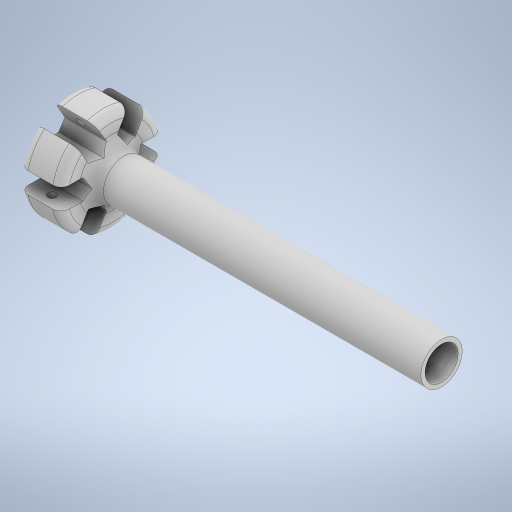
# Autodesk Inventor part: tija_suport
Saved by Autodesk Inventor 2024.2 (Build 282272000, 272)
## iProperties
Created: 2024-03-13
Part Number: tija_suport
Material: Genérico
Document SubType Name: Modeling
Designer: riera
Density: 1 g/cm^3
Appearance: Valor por defecto
Author: riera
Autodesk Inventor part; units mm, degrees
ref_plane "YZ Plane" through (0, 0, 0) normal (1, 0, 0) x (0, 1, 0)
ref_plane "XY Plane" through (0, 0, 0) normal (0, 0, 1) x (1, 0, 0)
sketch "Boceto1" plane through (0, 0, 0) normal (1, 0, 0) x (0, 1, 0)
  circle A0 centre (0, 0) radius 12.5
  dimension "d0" = 25
  constraints: 1 centre point, 1 coincident
  measures "d0" diameter of A0
extrude "Extrusión1" add sketch "Boceto1" along normal blind 10
sketch "Boceto2" plane through (10, 0, 0) normal (1, 0, 0) x (0, 0, -1)
  circle A0 centre (0, 0) radius 5
  circle A1 centre (0, 0) radius 4
  dimension "d3" = 10
  dimension "d35" = 8
  constraints: 2 centre point, 2 coincident
  measures "d3" diameter of A0
  measures "d35" diameter of A1
extrude "Extrusión2" add sketch "Boceto2" along normal blind 80
sketch "Boceto3" plane through (0, 0, 0) normal (-1, 0, 0) x (0, 0, 1)
  circle A0 centre (0, 0) radius 12.5 projected
  line L0 (6.9974, 2.5) -> (5.7474, 0)
  line L1 (5.7474, 0) -> (6.9974, -2.5)
  line L2 (0, 0) -> (0, 7.6455)
  line L3 (6.9974, 2.5) -> (12.5, 2.5)
  line L4 (6.9974, -2.5) -> (12.5, -2.5)
  line L5 (12.5, -2.5) -> (12.5, 2.5)
  dimension "d9" = 1.25
  dimension "d12" = 5.7474
  constraints: 12 end point, 2 horizontal, 1 perpendicular, 1 vertical
  measures "d9" horizontal distance of L1.end L0.end
  measures "d12" distance of L0.end point (0, 0)
extrude "Extrusión3" cut sketch "Boceto3" against normal blind 10 contours A0 L4 L1 L0 L3 | L5 L4 A0 | A0 L3 L5 picked at (8.8316, 0)
pattern_circular "Patrón circular1" count 6 over 360 about axis through (-10, 0, 0) along (1, 0, 0) of "Extrusión3"
fillet "Empalme1" radius 2 2 edges at (0, -6.25, -10.8253) (10, -6.25, -10.8253)
fillet "Empalme2" radius 2 10 edges at (0, 6.25, -10.8253) (10, 6.25, -10.8253) (0, -12.5, 0) (10, -12.5, 0) (0, -6.25, 10.8253) (10, -6.25, 10.8253) (10, 12.5, 0) (0, 12.5, 0) (0, 6.25, 10.8253) (10, 6.25, 10.8253)
sketch "Boceto4" plane through (0, 0, 0) normal (0, 1, 0) x (-1, 0, 0)
  line L0 (-8, -12.2474) -> (-2, -12.2474) projected
  line L1 (0, -10.198) -> (0, -6.9974) projected
  line L2 (0, -6.9974) -> (0, -5.7474) projected
  line L3 (0, -6.9974) -> (-10, -6.9974) projected
  line L4 (-10, -5.7474) -> (-10, -6.9974) projected
  line L5 (0, -5.7474) -> (-10, -5.7474) projected
  circle A0 centre (-5, -9.7474) radius 1
  point P0 (0, 0)
  point P1 (-5, -12.2474)
  dimension "d29" = 2
  dimension "d30" = 2.5
  dimension "d31" = 4
  constraints: 1 centre point, 1 midpoint
  measures "d29" diameter of A0
  measures "d30" distance of point (-5, -12.247) A0.centre
  measures "d31" distance from line of L5 A0.centre
ref_plane "Plano de trabajo1" through (0, 0, 0) normal (0, 1, 0) x (-1, 0, 0)
sketch "Boceto5" plane through (0, 0, 0) normal (0, 1, 0) x (-1, 0, 0)
  line L0 (6.5014, 0) -> (-26.2928, 0)
  point P0 (0, 0)
  constraints: 2 end point, 1 horizontal
revolve "Revolución1" cut sketch "Boceto4" angle 360 mid plane about axis through (-6.5014, 0, 0) along (1, 0, 0) contours A0
fillet "Empalme3" radius 3 1 edges at (10, 0, 5)
